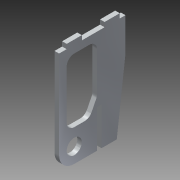
# Autodesk Inventor part: OpenROV 2_3 Dev Handle1
Saved by Autodesk Inventor 2013 (Build 170138000, 138)
## iProperties
Created: 2011-12-01
Part Number: OpenROV 2_3 Dev Handle1
Document SubType Name: Modeling
Designer: user
Density: 1 g/cm^3
Material: Generic
Author: user
Autodesk Inventor part; units mm, degrees
ref_plane "YZ Plane" through (0, 0, 0) normal (1, 0, 0) x (0, 1, 0)
ref_plane "XZ Plane" through (0, 0, 0) normal (0, 1, 0) x (-1, 0, 0)
ref_plane "XY Plane" through (0, 0, 0) normal (0, 0, 1) x (1, 0, 0)
sketch "Sketch1" plane through (0, 0, 0) normal (0, 0, 1) x (1, 0, 0)
  line L0 (15.75, -68) -> (15.75, -43)
  line L1 (15.75, -43) -> (18.75, -43)
  line L2 (18.75, -43) -> (18.75, -68)
  line L3 (43.75, -58) -> (43.75, 0)
  arc A0 (33.75, -68) -> (43.75, -58) centre (33.75, -58) ccw
  circle A1 centre (33.75, -58) radius 5
  line L4 (13.75, 0) -> (13.75, 3)
  line L5 (13.75, 3) -> (3.75, 3)
  line L6 (3.75, 3) -> (3.75, 0)
  line L7 (28.75, 0) -> (28.75, 3)
  line L8 (28.75, 3) -> (38.75, 3)
  line L9 (38.75, 3) -> (38.75, 0)
  line L10 (43.75, 0) -> (38.75, 0)
  line L11 (28.75, 0) -> (13.75, 0)
  line L12 (3.75, 0) -> (0, 0)
  line L13 (0, 0) -> (0, -21.8755)
  line L14 (5.75, -68) -> (0.0154, -22.1236)
  arc A2 (0, -21.8755) -> (0.0154, -22.1236) centre (2, -21.8755) ccw
  line L15 (33.75, -68) -> (18.75, -68)
  line L16 (15.75, -68) -> (5.75, -68)
  line L17 (26.8402, -47) -> (33.75, -47)
  line L18 (38.75, -42) -> (38.75, -10)
  line L19 (22.368, -44.2361) -> (19.2779, -38.0557)
  line L20 (33.75, -5) -> (23.75, -5)
  line L21 (18.75, -10) -> (18.75, -35.8197)
  arc A3 (23.75, -5) -> (18.75, -10) centre (23.75, -10) ccw
  arc A4 (38.75, -10) -> (33.75, -5) centre (33.75, -10) ccw
  arc A5 (33.75, -47) -> (38.75, -42) centre (33.75, -42) ccw
  arc A6 (22.368, -44.2361) -> (26.8402, -47) centre (26.8402, -42) ccw
  arc A7 (18.75, -35.8197) -> (19.2779, -38.0557) centre (23.75, -35.8197) ccw
  point P0 (43.75, -69.5)
  point P1 (0, -22)
  point P2 (23.75, -47)
  point P3 (18.75, -37)
  dimension "d7" = 10
  dimension "d12" = 10
  dimension "d17" = 10
  dimension "d18" = 3
  dimension "d20" = 10
  dimension "d21" = 3
  dimension "d22" = 5
  dimension "d23" = 15
  dimension "d24" = 3
  dimension "d25" = 3
  dimension "d42" = 3
  dimension "d46" = 3.75
  dimension "d47" = 22
  dimension "d49" = 2
  dimension "d54" = 10
  dimension "d55" = 15
  dimension "d57" = 68
  dimension "d58" = 15.75
  dimension "d59" = 25
  dimension "d61" = 5
  dimension "d65" = 5
  dimension "d66" = 10
  dimension "d67" = 5
  dimension "d68" = 5
  constraints: 44 end point, 15 tangent, 14 point on circle, 8 centre point, 7 point on line, 4 equal radius, 4 perpendicular, 2 parallel, 1 coincident
  measures "d7" radius of A0
  measures "d12" diameter of A1
  measures "d17" distance of L4.end L5.end
  measures "d18" distance of L5.end L6.end
  measures "d20" distance of L7.end L8.end
  measures "d21" distance of L8.end L9.end
  measures "d22" distance between parallel lines of L3 L9
  measures "d23" distance of L7.start L4.start
  measures "d24" distance of L4.start L4.end
  measures "d25" distance of L7.start L7.end
  measures "d42" distance between parallel lines of L0 L2
  measures "d46" distance between parallel lines of L13 L6
  measures "d47" distance of L12.end point (0, -22)
  measures "d49" radius of A2
  measures "d54" distance of L0.start L14.start
  measures "d55" distance of L15.start L2.end
  measures "d57" distance between parallel lines of L16 L12
  measures "d58" distance between parallel lines of L13 L0
  measures "d59" distance between parallel lines of L16 L1
  measures "d61" distance between parallel lines of L3 L18
  measures "d65" distance from line of point (23.75, -47) L2
  measures "d66" distance from line of L17 point (18.75, -37)
  measures "d67" radius of A3
  measures "d68" distance between parallel lines of L11 L20
extrude "Extrusion2" add sketch "Sketch1" along normal blind 3
body "Solid2"
